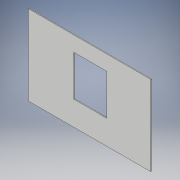
# Autodesk Inventor part: NorthWall
Saved by Autodesk Inventor 2018 (Build 220112000, 112)
## iProperties
Created: 2019-04-28
Part Number: NorthWall
Material: Generic
Document SubType Name: Modeling
Designer: snipe
Density: 1 g/cm^3
Appearance: Default
Author: snipe
Autodesk Inventor part; units mm, degrees
ref_plane "YZ Plane" through (0, 0, 0) normal (1, 0, 0) x (0, 1, 0)
ref_plane "XZ Plane" through (0, 0, 0) normal (0, 1, 0) x (-1, 0, 0)
ref_plane "XY Plane" through (0, 0, 0) normal (0, 0, 1) x (1, 0, 0)
sketch "Sketch1" plane through (0, 0, 0) normal (0, 0, 1) x (1, 0, 0)
  line L0 (0, 1813.56) -> (0, -1813.56) projected
  line L1 (-2773.68, 0) -> (2773.68, 0) projected
  line L2 (0, -1813.56) -> (0, 1813.56) projected
  line L3 (-2773.68, 0) -> (2773.68, 0) projected
  line L4 (-1981.2, -1295.4) -> (1981.2, -1295.4)
  line L5 (1981.2, -1295.4) -> (1981.2, 1295.4)
  line L6 (1981.2, 1295.4) -> (-1981.2, 1295.4)
  line L7 (-1981.2, 1295.4) -> (-1981.2, -1295.4)
  point P0 (0, 0)
  dimension "d0" = 3962.4
  dimension "d1" = 2590.8
  constraints: 8 end point, 2 parallel, 1 horizontal, 1 perpendicular, 2 other
  measures "d0" distance of L6.end L5.end
  measures "d1" distance of L5.end L4.end
extrude "Extrusion1" add sketch "Sketch1" along normal blind 25.4
sketch "Sketch2" plane through (0, 0, 25.4) normal (0, 0, 1) x (1, 0, 0)
  line L0 (-1981.2, -1295.4) -> (1981.2, -1295.4) projected
  line L1 (1981.2, -1295.4) -> (1981.2, 1295.4) projected
  line L2 (1981.2, 1295.4) -> (-1981.2, 1295.4) projected
  line L3 (-1981.2, 1295.4) -> (-1981.2, -1295.4) projected
  line L4 (1981.2, 1295.4) -> (-1981.2, 1295.4) projected
  line L5 (-1981.2, -1295.4) -> (-558.8, -1295.4)
  line L6 (-558.8, -1295.4) -> (-558.8, 1295.4)
  line L7 (-558.8, 1295.4) -> (-1981.2, 1295.4)
  line L8 (-1981.2, 1295.4) -> (-1981.2, -1295.4)
  line L9 (1981.2, -1295.4) -> (609.6, -1295.4)
  line L10 (609.6, -1295.4) -> (609.6, 1295.4)
  line L11 (609.6, 1295.4) -> (1981.2, 1295.4)
  line L12 (1981.2, 1295.4) -> (1981.2, -1295.4)
  line L13 (-558.8, 1295.4) -> (-508, 1295.4)
  line L14 (-508, 1295.4) -> (-508, -1295.4)
  line L15 (-508, -1295.4) -> (-558.8, -1295.4)
  line L16 (-558.8, -1295.4) -> (-558.8, 1295.4)
  line L17 (609.6, -1295.4) -> (558.8, -1295.4)
  line L18 (558.8, -1295.4) -> (558.8, 1295.4)
  line L19 (558.8, 1295.4) -> (609.6, 1295.4)
  line L20 (609.6, 1295.4) -> (609.6, -1295.4)
  line L21 (-508, 1295.4) -> (558.8, 1295.4)
  line L22 (558.8, 1295.4) -> (558.8, -1295.4)
  line L23 (558.8, -1295.4) -> (-508, -1295.4)
  line L24 (-508, -1295.4) -> (-508, 1295.4)
  line L25 (-508, 1295.4) -> (558.8, 1295.4)
  line L26 (558.8, 1295.4) -> (558.8, 889)
  line L27 (558.8, 889) -> (-508, 889)
  line L28 (-508, 889) -> (-508, 1295.4)
  line L29 (-508, 889) -> (-406.4, 889)
  line L30 (-508, 592.1375) -> (-508, 889)
  line L31 (-508, 889) -> (558.8, 889)
  line L32 (558.8, 889) -> (558.8, 812.8)
  line L33 (558.8, 812.8) -> (-508, 812.8)
  line L34 (-508, 812.8) -> (-508, 889)
  line L35 (-508, 812.8) -> (558.8, 812.8)
  line L36 (558.8, 812.8) -> (558.8, -508)
  line L37 (558.8, -508) -> (-508, -508)
  line L38 (-508, -508) -> (-508, 812.8)
  point P0 (0, 0)
  dimension "d4" = 1422.4
  dimension "d5" = 1371.6
  dimension "d6" = 50.8
  dimension "d7" = 50.8
  dimension "d8" = 406.4
  dimension "d10" = 76.2
  dimension "d11" = 1320.8
  constraints: 68 end point, 16 parallel, 9 horizontal, 8 perpendicular, 7 point on line
  measures "d4" distance of L7.end L6.end
  measures "d5" distance of L10.end L11.end
  measures "d6" distance of L14.end L15.end
  measures "d7" distance of L18.end L19.end
  measures "d8" distance of L25.end L26.end
  measures "d10" distance of L31.end L32.end
  measures "d11" distance of L35.end L36.end
extrude "Extrusion2" cut sketch "Sketch2" against normal blind 25.4 contours L14 L33 L18 L37
body "Solid1"
